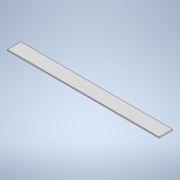
# Autodesk Inventor part: Plate8_80_1000
Saved by Autodesk Inventor 2020.1 (Build 241239000, 239)
## iProperties
Created: 2023-01-06
Part Number: Plate8_80_1000
Material: Типовые
Document SubType Name: Modeling
Designer: KirikDK
Mass: 1600 g
Surface Area: 3432 cm^2
Volume: 1600 cm^3
Density: 1 g/cm^3
Appearance: По умолчанию
Author: KirikDK
Autodesk Inventor part; units mm, degrees
ref_plane "YZ Plane" through (0, 0, 0) normal (1, 0, 0) x (0, 1, 0)
ref_plane "XZ Plane" through (0, 0, 0) normal (0, 1, 0) x (-1, 0, 0)
ref_plane "XY Plane" through (0, 0, 0) normal (0, 0, 1) x (1, 0, 0)
sketch "Эскиз1" plane through (0, 0, 0) normal (0, 1, 0) x (-1, 0, 0)
  line L0 (29.4072, 36.759) -> (-970.5928, 36.759)
  line L1 (-970.5928, 36.759) -> (-970.5928, -51.241)
  line L2 (-970.5928, -51.241) -> (29.4072, -51.241)
  line L3 (29.4072, -51.241) -> (29.4072, 36.759)
  point P0 (0, 0)
  dimension "d0" = 88
  dimension "d1" = 1000
  constraints: 8 end point, 2 parallel, 1 horizontal, 1 perpendicular
  measures "d0" distance of L2.end L0.start
  measures "d1" distance of L0.start L0.end
extrude "Выдавливание1" add sketch "Эскиз1" along normal blind 8
